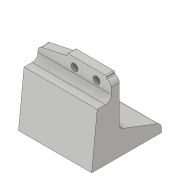
# Autodesk Inventor part: Part2
Saved by Autodesk Inventor 2018 (Build 220112000, 112)
## iProperties
Created: 2017-05-24
Part Number: Part2
Material: Generic
Document SubType Name: Modeling
Designer: anand
Density: 1 g/cm^3
Appearance: Default
Author: anand
Autodesk Inventor part; units mm, degrees
ref_plane "YZ Plane" through (0, 0, 0) normal (1, 0, 0) x (0, 1, 0)
ref_plane "XZ Plane" through (0, 0, 0) normal (0, 1, 0) x (-1, 0, 0)
ref_plane "XY Plane" through (0, 0, 0) normal (0, 0, 1) x (1, 0, 0)
sketch "Sketch2" plane through (0, 0, 0) normal (1, 0, 0) x (0, 1, 0)
  line L0 (0, 0) -> (0, -30.48)
  line L1 (0, -30.48) -> (3.556, -30.48)
  line L2 (3.556, -30.48) -> (10.6288, -12.0547)
  line L3 (10.6288, -12.0547) -> (30.48, -12.0547)
  line L4 (30.48, -12.0547) -> (30.48, -8.4987)
  line L5 (30.48, -8.4987) -> (22.86, -8.4987)
  line L6 (22.86, -8.4987) -> (22.86, -2.4027)
  line L7 (22.86, -2.4027) -> (0, 0)
  dimension "d0" = 30.48
  dimension "d1" = 21
  dimension "d2" = 84
  dimension "d3" = 30.48
  dimension "d4" = 22.86
  dimension "d5" = 3.556
  dimension "d6" = 9.652
  dimension "d7" = 3.556
  constraints: 16 end point, 4 perpendicular, 1 parallel, 1 vertical
  measures "d0" distance of L0.start L0.end
  measures "d1" angle of L0 L2
  measures "d2" angle of L0 L7
  measures "d3" distance between parallel lines of L0 L4
  measures "d4" distance between parallel lines of L6 L0
  measures "d5" distance of L3.end L4.end
  measures "d6" distance from line of L3 L6.end
  measures "d7" distance of L0.end L1.end
extrude "Extrusion1" add sketch "Sketch2" along normal mid plane 32.004
sketch "Sketch3" plane through (-16.002, 22.86, -8.4987) normal (0, 0, 1) x (1, 0, 0)
  line L0 (0, 7.62) -> (0, -12.2312) projected
  line L1 (0, 7.62) -> (12.7, 7.62)
  line L2 (0, 7.62) -> (32.004, 7.62) projected
  line L3 (0, 4.9205) -> (0, 7.62)
  line L4 (0, 4.9205) -> (12.7, 7.62)
  point P0 (16.002, -22.86)
  dimension "d10" = 12
  dimension "d11" = 12.7
  constraints: 6 end point, 1 point on line, 1 vertical
  measures "d10" angle of L4 L1
  measures "d11" distance of L0.start L1.end
extrude "Extrusion2" cut sketch "Sketch3" against normal blind 32.004
sketch "Sketch4" plane through (-16.002, 22.86, -8.4987) normal (0, 0, 1) x (1, 0, 0)
  line L0 (0, 4.9205) -> (12.7, 7.62) projected
  line L1 (12.7, 7.62) -> (29.972, 7.62)
  line L2 (29.972, 7.62) -> (29.972, 8.636)
  line L3 (29.972, 8.636) -> (12.7, 8.636)
  line L4 (12.7, 8.636) -> (12.7, 7.62)
  line L5 (32.004, 7.62) -> (32.004, 0) projected
  point P0 (16.002, -22.86)
  dimension "d15" = 1.016
  dimension "d18" = 17.272
  constraints: 8 end point, 2 parallel, 1 horizontal, 1 perpendicular
  measures "d15" distance of L1.end L2.end
  measures "d18" distance of L2.end L3.end
extrude "Extrusion3" add sketch "Sketch4" against normal up to surface (3.556 mm away)
fillet "Fillet1" radius 2.54 1 edges at (0, 22.86, -8.4987)
fillet "Fillet2" radius 2.032 1 edges at (-16.002, 27.7805, -10.2767)
fillet "Fillet3" radius 2.54 1 edges at (16.002, 30.48, -10.2767)
fillet "Fillet4" radius 2.032 1 edges at (0, 10.6288, -12.0547)
fillet "Fillet4" radius 2.54 1 edges at (0, 3.556, -30.48)
fillet "Fillet4" radius 0.508 4 edges at (13.97, 30.48, -10.2767) (13.97, 31.496, -10.2767) (-3.302, 31.496, -10.2767) (-3.302, 30.48, -10.2767)
sketch "Sketch5" plane through (-16.002, 22.86, -8.4987) normal (0, 0, 1) x (1, 0, 0)
  line L0 (0, 0) -> (32.004, 0) projected
  line L1 (32.004, 7.62) -> (32.004, 0) projected
  point P0 (16.002, -22.86)
  point P1 (16.002, 4.826)
  point P2 (25.654, 4.826)
  dimension "d28" = 9.652
  dimension "d29" = 4.826
  dimension "d30" = 6.35
  constraints: 1 horizontal alignment
  measures "d28" distance of point (25.654, 4.826) point (16.002, 4.826)
  measures "d29" distance from line of L0 point (25.654, 4.826)
  measures "d30" distance from line of L1 point (25.654, 4.826)
hole "Hole2" at (0, 27.686, -8.4987) at (9.652, 27.686, -8.4987) direction (0, 0, -1) diameter 3.048 end through all
body "Solid1"
